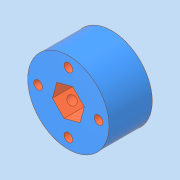
# Autodesk Inventor part: HexNutShaftServoCoupler
Saved by Autodesk Inventor 2017.3 (Build 213256000, 256)
## iProperties
Created: 2018-07-01
Part Number: HexNutShaftServoCoupler
Material: ABS Plastic
Document SubType Name: Modeling
Designer: Derek Wider
Density: 1.06 g/cm^3
Appearance: Smooth - White(2)
Author: Derek Wider
Autodesk Inventor part; units mm, degrees
ref_plane "YZ Plane" through (0, 0, 0) normal (1, 0, 0) x (0, 1, 0)
ref_plane "XZ Plane" through (0, 0, 0) normal (0, 1, 0) x (-1, 0, 0)
ref_plane "XY Plane" through (0, 0, 0) normal (0, 0, 1) x (1, 0, 0)
sketch "Sketch1" plane through (0, 0, 0) normal (0, 0, 1) x (1, 0, 0)
  circle A0 centre (0, 0) radius 11.938
  dimension "d0" = 23.876
  constraints: 1 centre point, 1 coincident
  measures "d0" diameter of A0
extrude "Extrusion1" add sketch "Sketch1" along normal blind 12.7
sketch "Sketch3" plane through (0, 0, 0) normal (0, 0, -1) x (-1, 0, 0)
  circle A0 centre (8.89, 0) radius 1.27
  circle A1 centre (0, 8.89) radius 1.27
  circle A2 centre (-8.89, 0) radius 1.27
  circle A3 centre (0, -8.89) radius 1.27
  point P0 (0, 0)
  dimension "d3" = 2.54
  dimension "d4" = 8.89
  dimension "d7" = 360
  constraints: 4 centre point, 9 other
  measures "d3" diameter of A0
  measures "d4" distance of point (0, 0) A0.centre
extrude "Extrusion2" cut sketch "Sketch3" against normal through all
sketch "Sketch4" plane through (0, 0, 12.7) normal (0, 0, 1) x (1, 0, 0)
  line L0 (4.6745, 1.2525) -> (3.4219, -3.4219)
  line L1 (3.4219, -3.4219) -> (-1.2525, -4.6745)
  line L2 (-1.2525, -4.6745) -> (-4.6745, -1.2525)
  line L3 (-4.6745, -1.2525) -> (-3.4219, 3.4219)
  line L4 (-3.4219, 3.4219) -> (1.2525, 4.6745)
  line L5 (1.2525, 4.6745) -> (4.6745, 1.2525)
  circle A0 centre (8.89, 0) radius 1.27 projected
  circle A1 centre (-8.89, 0) radius 1.27 projected
  circle A2 centre (0, 8.89) radius 1.27 projected
  circle A3 centre (0, -8.89) radius 1.27 projected
  circle A4 centre (0, 0) radius 11.938 projected
  line L6 (-2.9635, -2.9635) -> (-8.4414, -8.4414) construction
  circle A5 centre (0, 0) radius 11.938 construction
  line L7 (-8.89, 0) -> (-8.4414, -8.4414) construction
  line L8 (0, -8.89) -> (-8.4414, -8.4414) construction
  dimension "d11" = 8.382
  constraints: 18 end point, 1 coincident, 1 equal length, 1 midpoint, 1 perpendicular, 15 other
  measures "d11" distance between parallel lines of L4 L1
extrude "Extrusion3" cut sketch "Sketch4" against normal blind 7.62 contours L0 L1 L2 L3 L4 L5
sketch "Sketch5" plane through (0, 0, 0) normal (0, 0, -1) x (-1, 0, 0)
  circle A0 centre (0, 0) radius 2.54
  dimension "d14" = 5.08
  constraints: 1 centre point, 1 coincident
  measures "d14" diameter of A0
extrude "Extrusion4" cut sketch "Sketch5" against normal through all
sketch "Sketch7" plane through (-1.2525, -4.6745, 5.08) normal (0.7071068, 0.7071068, 0) x (-0.7071068, 0.7071068, 0)
  circle A0 centre (2.4197, 3.556) radius 1.2688
  line L0 (14.3577, 7.62) -> (-9.5183, 7.62) projected
  line L1 (13.5978, 7.62) -> (13.5978, -5.08) construction
  line L2 (13.5978, -5.08) -> (-8.7585, -5.08) construction
  line L3 (-8.7585, -5.08) -> (-8.7585, 7.62) construction
  line L4 (-8.7585, 7.62) -> (0, 7.62) construction
  line L5 (0, 7.62) -> (4.8393, 7.62) construction
  line L6 (4.8393, 7.62) -> (13.5978, 7.62) construction
  line L7 (0, 7.62) -> (0, 0) construction
  line L8 (0, 0) -> (4.8393, 0) construction
  line L9 (4.8393, 0) -> (4.8393, 7.62) construction
  line L10 (13.5978, 7.62) -> (2.4197, 3.556) construction
  line L11 (2.4197, 3.556) -> (-8.7585, 7.62) construction
  point P0 (2.4197, -5.08)
  dimension "d22" = 4.064
  constraints: 4 end point, 1 centre point, 1 equal length
  measures "d22" distance from line of L0 L10.end
extrude "Extrusion6" cut sketch "Sketch7" against normal through all
sketch "Sketch8" plane through (0, 0, 0) normal (0, 0, -1) x (-1, 0, 0)
  circle A0 centre (0, 0) radius 4.064
  dimension "d25" = 8.128
  constraints: 1 centre point, 1 coincident
  measures "d25" diameter of A0
extrude "Extrusion7" cut sketch "Sketch8" against normal blind 0.889
chamfer "Chamfer1" distance 1.524 angle 45 1 edges at (2.54, 0, 0.889)
body "Solid1"
